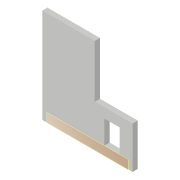
# Autodesk Inventor part: SensorWall
Saved by Autodesk Inventor 2018 (Build 220112000, 112)
## iProperties
Created: 2018-12-09
Part Number: SensorWall
Material: Generic
Document SubType Name: Modeling
Designer: ball
Density: 1 g/cm^3
Appearance: Default
Author: ball
Autodesk Inventor part; units mm, degrees
ref_plane "YZ Plane" through (0, 0, 0) normal (1, 0, 0) x (0, 1, 0)
ref_plane "XZ Plane" through (0, 0, 0) normal (0, 1, 0) x (-1, 0, 0)
ref_plane "XY Plane" through (0, 0, 0) normal (0, 0, 1) x (1, 0, 0)
ref_plane "Work Plane1" through (12, 156, 0) normal (0, 0, 1) x (0, -1, 0)
sketch "Sketch1" plane through (12, 156, 0) normal (0, 0, 1) x (0, -1, 0)
  line L0 (8, 72) -> (-36.75, 72) construction
  line L1 (-36.75, 72) -> (-36.5125, 72) construction
  line L2 (4, 64) -> (4, -8)
  line L3 (-36.75, 47.9255) -> (-36.75, 56.0811)
  line L4 (-88, -16) -> (4, -16)
  line L5 (4, -16) -> (4, 72)
  line L6 (4, 72) -> (-36.75, 72)
  line L7 (-88, 72) -> (-88.0072, 72)
  line L8 (-88.0072, 35.17) -> (-36.75, 35.17)
  line L9 (-36.75, 35.17) -> (-36.75, 72)
  line L10 (-27.25, 59.5) -> (-4.5297, 59.5)
  line L11 (-27.25, 46.6557) -> (-27.25, 50.4209)
  line L12 (-4.5297, 52.9092) -> (-4.5297, 57.2254)
  line L13 (-27.25, 44.5) -> (-4.5297, 44.5)
  line L14 (-4.5297, 44.5) -> (-4.5297, 59.5)
  line L15 (-4.5297, 59.5) -> (-27.25, 59.5)
  line L16 (-27.25, 59.5) -> (-27.25, 44.5)
  line L17 (-36.75, 44.5) -> (-36.75, 59.5)
  line L18 (-27.25, 59.5) -> (-27.25, 44.5)
  line L19 (-27.25, 59.5) -> (-4.5297, 59.5)
  line L20 (-4.5297, 59.5) -> (-4.5297, 44.5)
  line L21 (-4.5297, 44.5) -> (-27.25, 44.5)
  line L22 (-27.25, 44.5) -> (-27.25, 59.5)
  line L23 (-88, 35.17) -> (-88, -16)
  point P0 (156, -12)
  constraints: 48 end point, 8 parallel, 6 horizontal, 4 point on line, 4 vertical, 3 perpendicular, 11 other
extrude "Extrusion1" add sketch "Sketch1" against normal blind 5.08
body "Solid1"
